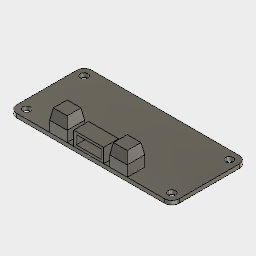
3346 Adafruit Speaker Bonnet for Pi (Autodesk Fusion 360 design; units mm, degrees)
Autodesk Fusion 360 part; units mm, degrees
sketch "PCB" plane through (0, 0, 0) normal (0, 0, 1) x (1, 0, 0)
  line L0 (0, 0) -> (65, 0)
  line L1 (65, 0) -> (65, 30)
  line L2 (65, 30) -> (0, 30)
  line L3 (0, 30) -> (0, 0)
  circle A0 centre (3.5, 3.5) radius 1.5
  line L4 (32.5, 30) -> (32.5, 0) construction
  line L5 (65, 15) -> (0, 15) construction
  circle A1 centre (61.5, 3.5) radius 1.5
  circle A2 centre (3.5, 26.5) radius 1.5
  circle A3 centre (61.5, 26.5) radius 1.5
  dimension "d1" = 65
  dimension "d2" = 30
  dimension "d3" = 3
  dimension "d4" = 3.5
  dimension "d5" = 3.5
  dimension "d13" = 58
  dimension "d14" = 23
  measures "d1" distance of L1.end L2.end
  measures "d2" distance of L0.end L1.end
  measures "d3" diameter of A0
  measures "d4" distance of L0 A0.centre
  measures "d5" distance of L3 A0.centre
extrude "Extrude1" add sketch "PCB" along normal blind 1.6 makes body 1
fillet "Fillet1" radius 3 4 edges at (0, 30, 0.8) (65, 30, 0.8) (0, 0, 0.8) (65, 0, 0.8) on bodies 1
sketch "Header" plane through (0, 0, 1.6) normal (0, 0, 1) x (-1, 0, 0)
  circle A0 centre (-3.5, -3.5) radius 1.5
  circle A1 centre (-61.5, -3.5) radius 1.5
  circle A2 centre (-61.5, -26.5) radius 1.5
  circle A3 centre (-3.5, -26.5) radius 1.5
  arc A4 (-62, 0) -> (-65, -3) centre (-62, -3) ccw
  line L0 (-65, -3) -> (-65, -27)
  arc A5 (-65, -27) -> (-62, -30) centre (-62, -27) ccw
  line L1 (-62, -30) -> (-3, -30)
  arc A6 (-3, -30) -> (0, -27) centre (-3, -27) ccw
  line L2 (0, -27) -> (0, -3)
  arc A7 (0, -3) -> (-3, 0) centre (-3, -3) ccw
  line L3 (-3, 0) -> (-62, 0)
  line L4 (-32.5, -30) -> (-32.5, 0) construction
  line L5 (-57.77, -24.2) -> (-7.23, -24.2)
  line L6 (-7.23, -24.2) -> (-7.23, -29.2)
  line L7 (-7.23, -29.2) -> (-57.77, -29.2)
  line L8 (-57.77, -29.2) -> (-57.77, -24.2)
  line L9 (-57.77, -24.2) -> (-7.23, -29.2) construction
  line L10 (-7.23, -24.2) -> (-57.77, -29.2) construction
  point P0 (-32.5, -26.7)
  dimension "d18" = 50.54
  dimension "d19" = 5
  dimension "d20" = 0.8
  measures "d18" distance of L6.end L7.end
  measures "d19" distance of L5.start L7.end
  measures "d20" distance of L1 L7
extrude "Extrude2" add sketch "Header" against normal blind 2.5 from surface at -1.6 separate body contours L5 L6 L7 L8 makes body 2
sketch "JST connector" plane through (0, 0, 1.6) normal (0, 0, 1) x (-1, 0, 0)
  circle A0 centre (-3.5, -3.5) radius 1.5
  circle A1 centre (-61.5, -3.5) radius 1.5
  circle A2 centre (-61.5, -26.5) radius 1.5
  circle A3 centre (-3.5, -26.5) radius 1.5
  arc A4 (-62, 0) -> (-65, -3) centre (-62, -3) ccw
  line L0 (-65, -3) -> (-65, -27)
  arc A5 (-65, -27) -> (-62, -30) centre (-62, -27) ccw
  line L1 (-62, -30) -> (-3, -30)
  arc A6 (-3, -30) -> (0, -27) centre (-3, -27) ccw
  line L2 (0, -27) -> (0, -3)
  arc A7 (0, -3) -> (-3, 0) centre (-3, -3) ccw
  line L3 (-3, 0) -> (-62, 0)
  line L4 (-25.75, 0) -> (-37.75, 0)
  line L5 (-37.75, 0) -> (-37.75, -8)
  line L6 (-37.75, -8) -> (-36.75, -8)
  line L7 (-36.75, -8) -> (-36.75, -6)
  line L8 (-36.75, -6) -> (-26.75, -6)
  line L9 (-26.75, -6) -> (-26.75, -8)
  line L10 (-26.75, -8) -> (-25.75, -8)
  line L11 (-25.75, -8) -> (-25.75, 0)
  line L12 (-31.75, 0) -> (-31.75, -6) construction
  dimension "d26" = 1
  dimension "d27" = 1
  dimension "d28" = 12
  dimension "d29" = 6
  dimension "d30" = 2
  dimension "d43" = 31.75
  measures "d26" distance of L9.end L10.end
  measures "d27" distance of L5.end L6.end
  measures "d28" distance of L4.start L4.end
  measures "d29" distance of L4 L8
  measures "d30" distance of L8.end L9.end
  measures "d43" distance of L2 L12
extrude "Extrude4" add sketch "JST connector" along normal blind 5.6 separate body contours L3 L4 L5 L6 L7 L8 L9 L10 L11 makes body 3
chamfer "Chamfer1" distance 2 angle 45 2 edges at (37.25, 8, 7.2) (26.25, 8, 7.2) on bodies 3
shell "Shell1" thickness 1 removed faces 1 at (29.75, 0, 3.4667) on bodies 3
sketch "termblocks" plane through (0, 0, 1.6) normal (0, 0, 1) x (-1, 0, 0)
  circle A0 centre (-3.5, -3.5) radius 1.5
  circle A1 centre (-61.5, -3.5) radius 1.5
  circle A2 centre (-61.5, -26.5) radius 1.5
  circle A3 centre (-3.5, -26.5) radius 1.5
  arc A4 (-62, 0) -> (-65, -3) centre (-62, -3) ccw
  line L0 (-65, -3) -> (-65, -27)
  arc A5 (-65, -27) -> (-62, -30) centre (-62, -27) ccw
  line L1 (-62, -30) -> (-3, -30)
  arc A6 (-3, -30) -> (0, -27) centre (-3, -27) ccw
  line L2 (0, -27) -> (0, -3)
  arc A7 (0, -3) -> (-3, 0) centre (-3, -3) ccw
  line L3 (-3, 0) -> (-62, 0)
  line L4 (-32.5, 0) -> (-32.5, -30) construction
  line L5 (-23.185, 0) -> (-16.185, 0)
  line L6 (-16.185, 0) -> (-16.185, -7)
  line L7 (-16.185, -7) -> (-23.185, -7)
  line L8 (-23.185, -7) -> (-23.185, 0)
  line L9 (-23.185, 0) -> (-16.185, -7) construction
  line L10 (-16.185, 0) -> (-23.185, -7) construction
  line L11 (-47.185, 0) -> (-40.185, 0)
  line L12 (-40.185, 0) -> (-40.185, -7)
  line L13 (-40.185, -7) -> (-47.185, -7)
  line L14 (-47.185, -7) -> (-47.185, 0)
  line L15 (-47.185, 0) -> (-40.185, -7) construction
  line L16 (-40.185, 0) -> (-47.185, -7) construction
  point P0 (-19.685, -3.5)
  point P1 (-43.685, -3.5)
  dimension "d35" = 7
  dimension "d36" = 7
  dimension "d37" = 19.685
  dimension "d40" = 7
  dimension "d41" = 7
  dimension "d42" = 24
  measures "d35" distance of L6.end L7.end
  measures "d36" distance of L5.end L6.end
  measures "d37" distance of L2 P0
  measures "d40" distance of L12.end L13.end
  measures "d41" distance of L11.end L12.end
  measures "d42" distance of P0 P1
extrude "Extrude5" add sketch "termblocks" along normal blind 4.25 separate body contours L3 L11 L12 L13 L14 | L3 L5 L6 L7 L8 makes body 4 at (20.8517, 2.3333, 1.6) makes body 5 at (44.8517, 2.3333, 1.6)
sketch "topblocks" plane through (0, 0, 5.85) normal (0, 0, 1) x (-1, 0, 0)
  line L0 (-23.185, -7) -> (-16.185, -7)
  line L1 (-16.185, -7) -> (-16.185, 0)
  line L2 (-16.185, 0) -> (-23.185, 0)
  line L3 (-23.185, 0) -> (-23.185, -7)
  line L4 (-47.185, -7) -> (-40.185, -7)
  line L5 (-40.185, -7) -> (-40.185, 0)
  line L6 (-40.185, 0) -> (-47.185, 0)
  line L7 (-47.185, 0) -> (-47.185, -7)
extrude "Extrude6" add sketch "topblocks" along normal blind 4.25 draft -10 bodies 4 5
equation "d38 = ( 8.5 / 2 ) * 1 mm"
equation "d44 = ( 8.5 / 2 ) * 1 mm"
named bodies: "PCB", "header", "JST", "left termblock", "right termblock"
